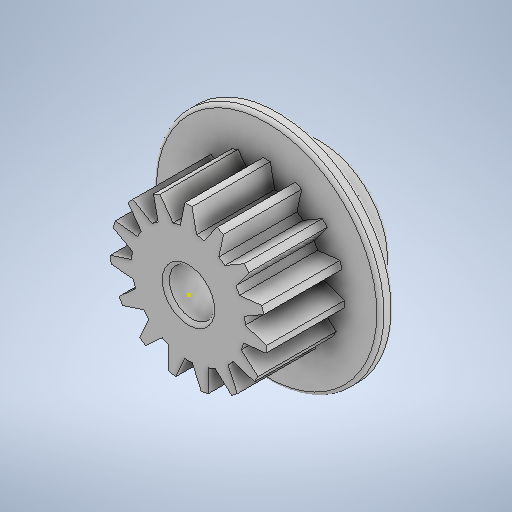
# Autodesk Inventor part: kolo_zebate_do_pasa_fi32_6,370_L19
Saved by Autodesk Inventor 2025.2 (Build 292293000, 293)
## iProperties
Created: 2025-03-20
Part Number: kolo_zebate_do_pasa_fi32_6,370_L19
Material: Ogólny
Document SubType Name: Modeling
Designer: rango
Density: 1 g/cm^3
Appearance: Domyślna
Author: rango
Autodesk Inventor part; units mm, degrees
ref_plane "YZ Plane" through (0, 0, 0) normal (1, 0, 0) x (0, 1, 0)
ref_plane "XZ Plane" through (0, 0, 0) normal (0, 1, 0) x (-1, 0, 0)
ref_plane "XY Plane" through (0, 0, 0) normal (0, 0, 1) x (1, 0, 0)
sketch "Szkic1" plane through (0, 0, 0) normal (0, 0, 1) x (1, 0, 0)
  circle A0 centre (0, 0) radius 9.5
  circle A1 centre (0, 0) radius 3.185
  dimension "d0" = 19
  dimension "d3" = 6.37
  constraints: 2 centre point, 2 coincident
  measures "d0" diameter of A0
  measures "d3" diameter of A1
extrude "Wyciągnięcie proste2" add sketch "Szkic1" along normal blind 6
sketch "Szkic2" plane through (0, 0, 6) normal (0, 0, 1) x (1, 0, 0)
  circle A0 centre (0, 0) radius 3.185 projected
  circle A1 centre (0, 0) radius 16
  circle A2 centre (0, 0) radius 3.185
  dimension "d6" = 32
  constraints: 2 centre point, 2 coincident
  measures "d6" diameter of A1
extrude "Wyciągnięcie proste3" add sketch "Szkic2" along normal blind 2
sketch "Szkic3" plane through (0, 0, 8) normal (0, 0, 1) x (1, 0, 0)
  circle A0 centre (0, 0) radius 8
  circle A1 centre (0, 0) radius 3.185
  line L0 (0, 8) -> (0, 11) construction
  line L1 (-0.5, 11) -> (0.5, 11)
  line L2 (0.5, 11) -> (1.1475, 7.9173)
  line L3 (-0.5, 11) -> (-1.1475, 7.9173)
  line L4 (-3.2539, 7.3084) -> (-4.4741, 10.049) construction
  line L5 (-4.9309, 9.8456) -> (-4.2686, 6.766)
  line L6 (-4.9309, 9.8456) -> (-4.0173, 10.2524)
  line L7 (-4.0173, 10.2524) -> (-2.1719, 7.6995)
  line L8 (-5.9452, 5.353) -> (-8.1746, 7.3604) construction
  line L9 (-8.5092, 6.9889) -> (-6.6515, 4.4449)
  line L10 (-8.5092, 6.9889) -> (-7.84, 7.732)
  line L11 (-7.84, 7.732) -> (-5.1158, 6.1505)
  line L12 (-7.6085, 2.4721) -> (-10.4616, 3.3992) construction
  line L13 (-10.6161, 2.9237) -> (-7.8844, 1.3552)
  line L14 (-10.6161, 2.9237) -> (-10.3071, 3.8747)
  line L15 (-10.3071, 3.8747) -> (-7.1752, 3.5379)
  line L16 (-7.9562, -0.8362) -> (-10.9397, -1.1498) construction
  line L17 (-10.8875, -1.6471) -> (-7.754, -1.9688)
  line L18 (-10.8875, -1.6471) -> (-10.992, -0.6526)
  line L19 (-10.992, -0.6526) -> (-7.9938, 0.3137)
  line L20 (-6.9282, -4) -> (-9.5263, -5.5) construction
  line L21 (-9.2763, -5.933) -> (-6.2828, -4.9524)
  line L22 (-9.2763, -5.933) -> (-9.7763, -5.067)
  line L23 (-9.7763, -5.067) -> (-7.4303, -2.9649)
  line L24 (-4.7023, -6.4721) -> (-6.4656, -8.8992) construction
  line L25 (-6.0611, -9.1931) -> (-3.7253, -7.0797)
  line L26 (-6.0611, -9.1931) -> (-6.8701, -8.6053)
  line L27 (-6.8701, -8.6053) -> (-5.582, -5.7307)
  line L28 (-1.6633, -7.8252) -> (-2.287, -10.7596) construction
  line L29 (-1.798, -10.8636) -> (-0.5236, -7.9828)
  line L30 (-1.798, -10.8636) -> (-2.7761, -10.6557)
  line L31 (-2.7761, -10.6557) -> (-2.7685, -7.5057)
  line L32 (1.6633, -7.8252) -> (2.287, -10.7596) construction
  line L33 (2.7761, -10.6557) -> (2.7685, -7.5057)
  line L34 (2.7761, -10.6557) -> (1.798, -10.8636)
  line L35 (1.798, -10.8636) -> (0.5236, -7.9828)
  line L36 (4.7023, -6.4721) -> (6.4656, -8.8992) construction
  line L37 (6.8701, -8.6053) -> (5.582, -5.7307)
  line L38 (6.8701, -8.6053) -> (6.0611, -9.1931)
  line L39 (6.0611, -9.1931) -> (3.7253, -7.0797)
  line L40 (6.9282, -4) -> (9.5263, -5.5) construction
  line L41 (9.7763, -5.067) -> (7.4303, -2.9649)
  line L42 (9.7763, -5.067) -> (9.2763, -5.933)
  line L43 (9.2763, -5.933) -> (6.2828, -4.9524)
  line L44 (7.9562, -0.8362) -> (10.9397, -1.1498) construction
  line L45 (10.992, -0.6526) -> (7.9938, 0.3137)
  line L46 (10.992, -0.6526) -> (10.8875, -1.6471)
  line L47 (10.8875, -1.6471) -> (7.754, -1.9688)
  line L48 (7.6085, 2.4721) -> (10.4616, 3.3992) construction
  line L49 (10.3071, 3.8747) -> (7.1752, 3.5379)
  line L50 (10.3071, 3.8747) -> (10.6161, 2.9237)
  line L51 (10.6161, 2.9237) -> (7.8844, 1.3552)
  line L52 (5.9452, 5.353) -> (8.1746, 7.3604) construction
  line L53 (7.84, 7.732) -> (5.1158, 6.1505)
  line L54 (7.84, 7.732) -> (8.5092, 6.9889)
  line L55 (8.5092, 6.9889) -> (6.6515, 4.4449)
  line L56 (3.2539, 7.3084) -> (4.4741, 10.049) construction
  line L57 (4.0173, 10.2524) -> (2.1719, 7.6995)
  line L58 (4.0173, 10.2524) -> (4.9309, 9.8456)
  line L59 (4.9309, 9.8456) -> (4.2686, 6.766)
  dimension "d9" = 16
  dimension "d10" = 3
  dimension "d11" = 1
  dimension "d12" = 3.15
  dimension "d15" = 360
  constraints: 120 end point, 2 coincident, 1 centre point, 1 horizontal, 1 vertical, 156 other
  measures "d10" distance of L0.start L0.end
  measures "d11" distance of L1.start L1.end
  measures "d12" distance of L1.end L2.end
extrude "Wyciągnięcie proste4" add sketch "Szkic3" along normal blind 11
sketch "Szkic4" plane through (0, 0, 19) normal (0, 0, 1) x (1, 0, 0)
  point P0 (0, 0)
fillet "Zaokrąglenie1" radius 0.5 1 edges at (-16, 0, 8)
fillet "Zaokrąglenie2" radius 0.5 4 edges at (-16, 0, 6) (-9.5, 0, 0) (-3.185, 0, 19) (-3.185, 0, 0)
